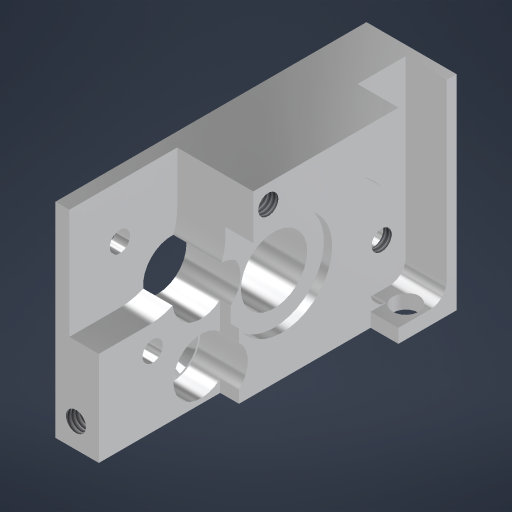
# Autodesk Inventor part: MocowaniePrawejPrzekladni
Saved by Autodesk Inventor 2023 (Build 270158000, 158)
## iProperties
Created: 2022-03-19
Part Number: MocowaniePrawejPrzekladni
Material: Aluminium 6061
Document SubType Name: Modeling
Designer: Michał
Density: 2.7 g/cm^3
Appearance: Aluminium — płaski
Mass: 13.7652 g
Surface Area: 41.6829 cm^2
Volume: 5.09822 cm^3
Author: Michał
Autodesk Inventor part; units mm, degrees
ref_plane "YZ Plane" through (0, 0, 0) normal (1, 0, 0) x (0, 1, 0)
ref_plane "XZ Plane" through (0, 0, 0) normal (0, 1, 0) x (-1, 0, 0)
ref_plane "XY Plane" through (0, 0, 0) normal (0, 0, 1) x (1, 0, 0)
sketch "Szkic1" plane through (0, 0, 0) normal (1, 0, 0) x (0, 1, 0)
  line L0 (0, 0) -> (25, 0)
  line L1 (25, 0) -> (25, -38)
  line L2 (25, -38) -> (0, -38)
  line L3 (0, -38) -> (0, 0)
  dimension "wysokosc" = 25
  dimension "dlugosc" = 38
  constraints: 8 end point, 2 parallel, 1 horizontal, 1 perpendicular
  measures "wysokosc" distance of L0.start L0.end
  measures "dlugosc" distance between parallel lines of L2 L0
extrude "Wyciągnięcie proste1" add sketch "Szkic1" along normal blind 11
sketch "Szkic2" plane through (11, 0, 0) normal (1, 0, 0) x (0, 0, -1)
  circle A0 centre (12.5, 12.5) radius 3.5
  line L0 (0, 25) -> (0, 0) projected
  line L1 (0, 0) -> (38, 0) projected
  circle A1 centre (6.1695, 18.5405) radius 1.25
  circle A2 centre (6.5703, 8.5486) radius 1.25
  circle A3 centre (20.1, 11) radius 4.05
  line L2 (38, 0) -> (38, 25) projected
  line L3 (38, 25) -> (0, 25) projected
  line L4 (30.9, 25) -> (36.8, 25)
  line L5 (36.8, 25) -> (36.8, 1.7)
  line L6 (36.8, 1.7) -> (30.9, 1.7)
  line L7 (30.9, 1.7) -> (30.9, 25)
  line L8 (6.5703, 8.5486) -> (20.1, 11) construction
  line L9 (20.1, 11) -> (20.1, 0) construction
  point P0 (15, 22.7)
  point P1 (33.85, 7)
  point P2 (33.85, 25)
  dimension "d4" = 7
  dimension "d5" = 12.5
  dimension "d6" = 12.5
  dimension "d7" = 2.5
  dimension "d8" = 8.1
  dimension "d9" = 11
  dimension "d10" = 20.1
  dimension "d12" = 8.75
  dimension "d13" = 10
  dimension "d14" = 13.75
  dimension "d54" = 7
  dimension "d55" = 23
  dimension "d56" = 2.3
  dimension "d64" = 1.7
  dimension "d65" = 33.85
  dimension "d66" = 5.9
  dimension "d102" = 100.27
  constraints: 12 end point, 4 centre point, 2 parallel, 2 perpendicular, 1 collinear, 1 equal radius, 1 horizontal, 1 midpoint, 1 point on line, 1 vertical alignment
  measures "d4" diameter of A0
  measures "d5" distance from line of L0 A0.centre
  measures "d6" distance from line of L1 A0.centre
  measures "d7" diameter of A1
  measures "d8" diameter of A3
  measures "d9" distance from line of L1 L8.end
  measures "d10" distance from line of L0 L8.end
  measures "d12" distance of A0.centre A1.centre
  measures "d13" distance of L8.start A1.centre
  measures "d14" distance of L8.end L8.start
  measures "d54" distance from line of L1 point (33.85, 7)
  measures "d55" distance from line of L2 point (15, 22.7)
  measures "d56" distance from line of L3 point (15, 22.7)
  measures "d64" distance between parallel lines of L1 L6
  measures "d65" distance from line of L0 point (33.85, 25)
  measures "d66" distance between parallel lines of L5 L7
  measures "d102" angle of L9 L8
extrude "Wyciągnięcie proste2" cut sketch "Szkic2" against normal through all contours A0 | A1 | A2 | A3
sketch "Szkic3" plane through (11, 0, 0) normal (1, 0, 0) x (0, 0, -1)
  circle A0 centre (12.5, 12.5) radius 3.5 projected
  line L0 (12.5, 12.5) -> (12.5, 4) construction
  line L1 (12.5, 12.5) -> (12.5, 21) construction
  point P0 (0, 0)
  dimension "d38" = 8.5
  constraints: 4 end point, 2 vertical, 1 collinear
  measures "d38" distance of L0.start L0.end
hole "Otwór4" at (11, 4, -12.5) direction (-1, 0, 0) diameter 6.8 depth 9.2
hole "Otwór1" at (11, 18.5405, -6.1695) direction (-1, 0, 0) diameter 14 depth 9.3
hole "Otwór2" at (11, 8.5486, -6.5703) direction (-1, 0, 0) diameter 16.5 depth 5.7
hole "Otwór3" at (11, 11, -20.1) direction (-1, 0, 0) diameter 22 depth 3.4
sketch "Szkic4" plane through (1.8, 21, -12.5) normal (1, 0, 0) x (0, 0, -1)
  circle A0 centre (0, -17) radius 3.4 construction
  point P0 (-12.5, -21)
  point P1 (0, 0)
  constraints: 1 coincident
hole "Otwór5" at (1.8, 4, -12.5) direction (-1, 0, 0) diameter 3.4 end through all countersink diameter 6.3 countersink angle 90 clearance for "Śruba ze łbem stożkowym ISO 2009/7046" size "M3" standard "ISO"
hole "Otwór6" at (11, 22.7, -15) at (11, 7, -33.85) direction (-1, 0, 0) diameter 2.459 depth 8.8 tip angle 118 thread size "M3x0.5" class "6H" standard "ISO Metric profile"
extrude "Wyciągnięcie proste3" cut sketch "Szkic2" against normal blind 5 contours L3 L5 L6 L7
sketch "Szkic5" plane through (0, 0, 0) normal (0, 0, 1) x (1, 0, 0)
  line L0 (0, 0) -> (0, 25) projected
  line L1 (0, 0) -> (11, 0) projected
  point P0 (2.5, 3)
  dimension "d39" = 6.8
  dimension "d69" = 2.5
  dimension "d70" = 3
  measures "d69" distance from line of L0 point (2.5, 3)
  measures "d70" distance from line of L1 point (2.5, 3)
hole "Otwór7" at (2.5, 3, 0) direction (0, 0, -1) diameter 2.459 depth 5 tip angle 118 thread size "M3x0.5" class "6H" standard "ISO Metric profile"
sketch "Szkic6" plane through (11, 0, 0) normal (1, 0, 0) x (0, 0, -1)
  arc A0 (0.6247, 14.268) -> (0, 13.5379) centre (6.5703, 8.5486) ccw projected
  arc A1 (0, 15.2335) -> (0.6247, 14.268) centre (6.1695, 18.5405) ccw projected
  line L0 (0, 15.2335) -> (0, 13.5379) projected
  point P0 (0, 0)
extrude "Wyciągnięcie proste4" cut sketch "Szkic6" against normal up to surface (5.7 mm away)
sketch "Szkic7" plane through (11, 1.7, -30.9) normal (0, 1, 0) x (1, 0, 0)
  line L0 (0, 0) -> (-3.4, 0) construction
  line L1 (-2.05, 0) -> (-2.05, 2.95) construction
  line L2 (-2.05, 2.95) -> (-5, 2.95) construction
  line L3 (-5, 0) -> (-5, 5.9) construction
  line L4 (-2.05, 2.95) -> (-2.05, 5.9) construction
  line L5 (-5, 5.9) -> (0, 5.9) construction
  point P0 (-11, -30.9)
  constraints: 6 end point, 3 point on line, 2 perpendicular, 1 horizontal, 1 midpoint, 1 vertical
hole "Otwór8" at (8.95, 1.7, -33.85) direction (0, -1, 0) diameter 3.2 end through all clearance for "Śruba ze łbem stożkowym ISO 2009/7046" size "M3" standard "ISO"
sketch "Szkic8" plane through (0, 0, -38) normal (0, 0, -1) x (-1, 0, 0)
  line L0 (0, 25) -> (0, 0) construction
  line L1 (0, 0) -> (-11, 0) construction
  point P0 (-2.5, 11)
  point P1 (-2.5, 21)
  dimension "d87" = 2.5
  dimension "d88" = 11
  dimension "d89" = 21
  constraints: 1 vertical alignment
  measures "d87" distance from line of L0 point (-2.5, 11)
  measures "d88" distance from line of L1 point (-2.5, 11)
  measures "d89" distance from line of point (-2.5, 21) L1
hole "Otwór9" at (2.5, 11, -38) at (2.5, 21, -38) direction (0, 0, 1) diameter 2.459 depth 6 tip angle 118 thread size "M3x0.5" class "6H" standard "ISO Metric profile"
sketch "Szkic9" plane through (0, 0, 0) normal (-1, 0, 0) x (0, 0, 1)
  line L0 (-20.1, 0) -> (-38, 0) projected
  line L1 (-38, 0) -> (-20, 0)
  line L2 (-20, 0) -> (-20, 4)
  line L3 (-20, 4) -> (-38, 4)
  line L4 (-38, 4) -> (-38, 0)
  line L5 (0, 0) -> (0, 25) projected
  dimension "d97" = 4
  dimension "d98" = 20
  constraints: 8 end point, 2 parallel, 1 horizontal, 1 perpendicular
  measures "d97" distance of L3.end L0.end
  measures "d98" distance between parallel lines of L2 L5
extrude "Wyciągnięcie proste5" cut sketch "Szkic9" against normal blind 2
fillet "Zaokrąglenie1" radius 2 1 edges at (1, 4, -20)
sketch "Szkic10" plane through (11, 0, 0) normal (1, 0, 0) x (0, 0, -1)
  arc A0 (3.4723, 25) -> (0, 21.8476) centre (6.1695, 18.5405) ccw projected
  line L0 (3.4723, 25) -> (0, 25) projected
  line L1 (0, 25) -> (0, 21.8476) projected
  line L2 (0, 0) -> (0, 25) projected
  line L3 (0, 21.8476) -> (0, 25)
  line L4 (0, 25) -> (3.4723, 25)
  line L5 (3.4723, 25) -> (8.8668, 25) projected
  arc A1 (3.4723, 25) -> (0, 21.8476) centre (6.1695, 18.5405) ccw projected
  line L6 (0, 15.2335) -> (0, 21.8476) projected
  arc A2 (0, 15.2335) -> (9.0179, 12.1462) centre (6.1695, 18.5405) ccw projected
  arc A3 (12.6902, 15.9948) -> (9.0179, 12.1462) centre (12.5, 12.5) ccw projected
  arc A4 (12.6902, 15.9948) -> (8.8668, 25) centre (6.1695, 18.5405) ccw projected
  circle A5 centre (6.1695, 18.5405) radius 1.25 projected
  line L7 (30.9, 25) -> (8.8668, 25) projected
  line L8 (13.1695, 25) -> (13.1695, 18.5405)
  arc A6 (13.1049, 19.4894) -> (8.8668, 25) centre (6.1695, 18.5405) ccw projected
  arc A7 (0, 15.2335) -> (9.0179, 12.1462) centre (6.1695, 18.5405) ccw projected
  line L9 (6.1695, 11.5405) -> (0, 11.5405)
  line L10 (8.8668, 25) -> (13.1695, 25)
  line L11 (0, 3.5592) -> (0, 15.2335) projected
  line L12 (0, 15.2335) -> (0, 11.5405)
  circle A8 centre (6.1695, 18.5405) radius 7
  line L13 (8.8668, 25) -> (13.1695, 25)
  arc A9 (12.6902, 15.9948) -> (8.8668, 25) centre (6.1695, 18.5405) ccw projected
  line L14 (13.1695, 18.5405) -> (8.8668, 25)
  constraints: 16 end point, 4 collinear, 3 point on line, 3 tangent, 2 perpendicular, 2 point on circle, 1 coincident, 1 vertical, 3 other
extrude "Wyciągnięcie proste6" cut sketch "Szkic10" against normal up to surface (9.3 mm away) contours L5 L14 A4 A3 A2 L2 A0 | A0 L1 L0 | L7 L8 A4 | A4 L14 | A2 L9 L2 | A5
sketch "Szkic13" plane through (11, 0, 0) normal (1, 0, 0) x (0, 0, -1)
  line L0 (6.1695, 11.5405) -> (0, 11.5405) projected
  line L1 (0, 3.5592) -> (0, 11.5405) projected
  arc A0 (0, 3.5592) -> (10.4654, 1.276) centre (6.5703, 8.5486) ccw projected
  arc A1 (14.6038, 6.671) -> (10.4654, 1.276) centre (12.5, 4) ccw projected
  arc A2 (14.6038, 6.671) -> (14.7251, 9.7983) centre (6.5703, 8.5486) ccw projected
  arc A3 (9.0179, 12.1462) -> (14.7251, 9.7983) centre (12.5, 12.5) ccw projected
  arc A4 (6.1695, 11.5405) -> (9.0179, 12.1462) centre (6.1695, 18.5405) ccw projected
  circle A5 centre (6.5703, 8.5486) radius 1.25 projected
  line L2 (20, 0) -> (0, 0) projected
  line L3 (0, 3.5592) -> (0, 11.5405) projected
  line L4 (0, 0) -> (0, 11.5405)
  line L5 (0, 11.5405) -> (14.8203, 11.5405)
  line L6 (14.8203, 11.5405) -> (14.8203, 0)
  line L7 (0, 0) -> (14.8203, 0)
  constraints: 8 end point, 2 perpendicular, 1 horizontal, 1 tangent, 1 vertical
extrude "Wyciągnięcie proste9" cut sketch "Szkic13" against normal up to surface (5.7 mm away)
sketch "Szkic14" plane through (11, 0, 0) normal (1, 0, 0) x (0, 0, -1)
  line L0 (14.8203, 1.5148) -> (14.8203, 1.3499) projected
  arc A0 (14.8203, 1.3499) -> (20.1, 0) centre (20.1, 11) ccw projected
  arc A1 (20.1, 0) -> (30.9, 8.9119) centre (20.1, 11) ccw projected
  line L1 (30.9, 8.9119) -> (30.9, 13.0881) projected
  arc A2 (30.9, 13.0881) -> (13.1695, 19.5422) centre (20.1, 11) ccw projected
  line L2 (13.1695, 19.5422) -> (13.1695, 18.5405) projected
  arc A3 (12.6902, 15.9948) -> (13.1695, 18.5405) centre (6.1695, 18.5405) ccw projected
  arc A4 (14.8203, 9.8797) -> (12.6902, 15.9948) centre (12.5, 12.5) ccw projected
  line L3 (14.8203, 9.8797) -> (14.8203, 6.4852) projected
  arc A5 (14.8203, 1.5148) -> (14.8203, 6.4852) centre (12.5, 4) ccw projected
  circle A6 centre (20.1, 11) radius 4.05 projected
  line L4 (30.9, 8.9119) -> (30.9, 0)
  line L5 (20.1, 0) -> (38, 0) projected
  line L6 (20.1, 0) -> (30.9, 8.9119)
  line L7 (30.9, 13.0881) -> (30.9, 25) projected
  line L8 (30.9, 13.0881) -> (30.9, 17.6)
  arc A7 (30.9, 13.0881) -> (13.1695, 19.5422) centre (20.1, 11) ccw projected
  line L9 (28.9, 17.6) -> (30.9, 13.0881)
  line L10 (28.9, 17.6) -> (30.9, 17.6)
  line L11 (14.8203, 0) -> (20.1, 0) projected
  line L12 (14.8203, 1.3499) -> (14.8203, 0)
  line L13 (14.8203, 0) -> (20.1, 0)
  point P0 (0, 0)
  dimension "d114" = 2
  constraints: 14 end point, 2 perpendicular, 2 point on line, 1 collinear, 1 point on circle, 1 vertical
  measures "d114" distance of L9.start L8.end
extrude "Wyciągnięcie proste10" cut sketch "Szkic14" against normal up to surface (3.4 mm away) contours A5 L3 A4 A3 L2 A2 L9 L1 L6 A0 L0 | A0 L11 L12 | A1 L4 L5 | L9 A2 | A2 L10 L7
fillet "Zaokrąglenie2" radius 2 2 edges at (8.5, 1.7, -36.8) (6.8, 1.7, -30.9)
sketch "Sketch15" plane through (7.6, 18.5405, -13.1695) normal (1, 0, 0) x (0, 0, -1)
  circle A0 centre (6.9305, -7.5405) radius 4.05 projected
  circle A1 centre (6.9305, -7.5405) radius 6.1
  point P0 (-13.1695, -18.5405)
  dimension "d118" = 12.2
  constraints: 1 centre point, 1 coincident
  measures "d118" diameter of A1
extrude "Extrusion11" cut sketch "Sketch15" against normal blind 1
